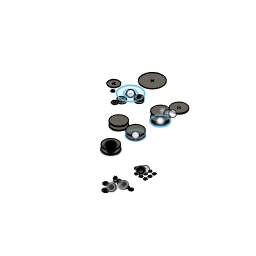
TwoBoardsThroghPlaneWith30mmHole v1 (Autodesk Fusion 360 design; units mm, degrees)
description: Spur Gear; Module: 2.0; Num Teeth: 16; Pressure Angle: 20.0; Backlash: 0.10 mm
Autodesk Fusion 360 part; units mm, degrees
(part 1 of 2)
sketch "Esquisse1" plane through (0, 0, 0) normal (0, 0, 1) x (1, 0, 0)
  circle A0 centre (0, 0) radius 70
  circle A1 centre (0, 0) radius 15
  dimension "d1" = 140
  dimension "d2" = 30
  constraint coincident A0.centre A1.centre
  constraint concentric A0 A1
  measures "d1" diameter of A0
  measures "d2" diameter of A1
sketch "Esquisse1 (2)" plane through (0, 0, 0) normal (0, 0, 1) x (1, 0, 0) in component "Spur Gear (16 teeth)"
  circle A0 centre (0, 0) radius 13.5492
  circle A1 centre (0, 0) radius 3
extrude "Extrusion1" add sketch "Esquisse1 (2)" along normal blind 2 contours A0 picked at (9.971186, -0.822177) makes body 1 in component "Spur Gear (16 teeth)"
sketch "Esquisse2" plane through (0, 0, 0) normal (0, 0, 1) x (1, 0, 0) in component "Spur Gear (16 teeth)"
  spline S0 degree 5 poles (14.941691, -1.673189) (14.950383, -1.674156) (14.967781, -1.675842) (14.993916, -1.677627) (15.028836, -1.678593) (15.072593, -1.677865) (15.116432, -1.675738) (15.160331, -1.672743) (15.204269, -1.669272) (15.248236, -1.665474) (15.292225, -1.661337) (15.336235, -1.656753) (15.380265, -1.651581) (15.424315, -1.645727) (15.468381, -1.639187) (15.512461, -1.632014) (15.556549, -1.624291) (15.600641, -1.616107) (15.644735, -1.607524) (15.688827, -1.598564) (15.732916, -1.589223) (15.777, -1.579481) (15.821079, -1.569317) (15.865151, -1.558721) (15.909214, -1.547697) (15.953267, -1.536261) (15.997307, -1.524432) (16.041334, -1.512231) (16.085345, -1.49967) (16.129338, -1.486758) (16.173313, -1.473495) (16.217269, -1.459883) (16.261203, -1.44592) (16.305115, -1.431607) (16.349004, -1.416949) (16.392868, -1.401951) (16.436706, -1.386619) (16.480518, -1.37096) (16.5243, -1.354979) (16.568053, -1.338679) (16.611776, -1.322063) (16.655467, -1.305134) (16.699125, -1.287892) (16.742749, -1.270341) (16.786339, -1.252484) (16.829892, -1.234323) (16.873409, -1.215861) (16.916887, -1.197102) (16.960326, -1.178048) (17.003726, -1.158702) (17.047084, -1.139066) (17.090401, -1.119141) (17.133674, -1.09893) (17.176904, -1.078435) (17.220089, -1.057658) (17.263228, -1.036601) (17.30632, -1.015266) (17.349365, -0.993655) (17.392361, -0.97177) (17.435308, -0.949612) (17.478204, -0.927183) (17.52105, -0.904486) (17.563844, -0.881521) (17.606585, -0.858289) (17.649272, -0.834794) (17.691904, -0.811036) (17.73448, -0.787018) (17.776999, -0.762741) (17.81946, -0.738205) (17.861864, -0.713414) (17.904209, -0.688366) (17.938038, -0.668124) (17.963384, -0.652828) (17.98027, -0.642579) (17.988709, -0.637443) knots 0 0 0 0 0 0 0.01428571 0.02857143 0.04285714 0.05714286 0.07142857 0.08571429 0.1 0.11428571 0.12857143 0.14285714 0.15714286 0.17142857 0.18571429 0.2 0.21428571 0.22857143 0.24285714 0.25714286 0.27142857 0.28571429 0.3 0.31428571 0.32857143 0.34285714 0.35714286 0.37142857 0.38571429 0.4 0.41428571 0.42857143 0.44285714 0.45714286 0.47142857 0.48571429 0.5 0.51428571 0.52857143 0.54285714 0.55714286 0.57142857 0.58571429 0.6 0.61428571 0.62857143 0.64285714 0.65714286 0.67142857 0.68571429 0.7 0.71428571 0.72857143 0.74285714 0.75714286 0.77142857 0.78571429 0.8 0.81428571 0.82857143 0.84285714 0.85714286 0.87142857 0.88571429 0.9 0.91428571 0.92857143 0.94285714 0.95714286 0.97142857 0.98571429 1 1 1 1 1 1
  spline S1 degree 5 poles (14.941691, 1.673189) (14.950383, 1.674156) (14.967781, 1.675842) (14.993916, 1.677627) (15.028836, 1.678593) (15.072593, 1.677865) (15.116432, 1.675738) (15.160331, 1.672743) (15.204269, 1.669272) (15.248236, 1.665474) (15.292225, 1.661337) (15.336235, 1.656753) (15.380265, 1.651581) (15.424315, 1.645727) (15.468381, 1.639187) (15.512461, 1.632014) (15.556549, 1.624291) (15.600641, 1.616107) (15.644735, 1.607524) (15.688827, 1.598564) (15.732916, 1.589223) (15.777, 1.579481) (15.821079, 1.569317) (15.865151, 1.558721) (15.909214, 1.547697) (15.953267, 1.536261) (15.997307, 1.524432) (16.041334, 1.512231) (16.085345, 1.49967) (16.129338, 1.486758) (16.173313, 1.473495) (16.217269, 1.459883) (16.261203, 1.44592) (16.305115, 1.431607) (16.349004, 1.416949) (16.392868, 1.401951) (16.436706, 1.386619) (16.480518, 1.37096) (16.5243, 1.354979) (16.568053, 1.338679) (16.611776, 1.322063) (16.655467, 1.305134) (16.699125, 1.287892) (16.742749, 1.270341) (16.786339, 1.252484) (16.829892, 1.234323) (16.873409, 1.215861) (16.916887, 1.197102) (16.960326, 1.178048) (17.003726, 1.158702) (17.047084, 1.139066) (17.090401, 1.119141) (17.133674, 1.09893) (17.176904, 1.078435) (17.220089, 1.057658) (17.263228, 1.036601) (17.30632, 1.015266) (17.349365, 0.993655) (17.392361, 0.97177) (17.435308, 0.949612) (17.478204, 0.927183) (17.52105, 0.904486) (17.563844, 0.881521) (17.606585, 0.858289) (17.649272, 0.834794) (17.691904, 0.811036) (17.73448, 0.787018) (17.776999, 0.762741) (17.81946, 0.738205) (17.861864, 0.713414) (17.904209, 0.688366) (17.938038, 0.668124) (17.963384, 0.652828) (17.98027, 0.642579) (17.988709, 0.637443) knots 0 0 0 0 0 0 0.01428571 0.02857143 0.04285714 0.05714286 0.07142857 0.08571429 0.1 0.11428571 0.12857143 0.14285714 0.15714286 0.17142857 0.18571429 0.2 0.21428571 0.22857143 0.24285714 0.25714286 0.27142857 0.28571429 0.3 0.31428571 0.32857143 0.34285714 0.35714286 0.37142857 0.38571429 0.4 0.41428571 0.42857143 0.44285714 0.45714286 0.47142857 0.48571429 0.5 0.51428571 0.52857143 0.54285714 0.55714286 0.57142857 0.58571429 0.6 0.61428571 0.62857143 0.64285714 0.65714286 0.67142857 0.68571429 0.7 0.71428571 0.72857143 0.74285714 0.75714286 0.77142857 0.78571429 0.8 0.81428571 0.82857143 0.84285714 0.85714286 0.87142857 0.88571429 0.9 0.91428571 0.92857143 0.94285714 0.95714286 0.97142857 0.98571429 1 1 1 1 1 1
  arc A0 (17.988709, -0.637443) -> (17.988709, 0.637443) centre (0, 0) ccw
  line L0 (13.455101, -1.507832) -> (14.941691, -1.673189)
  line L1 (13.455101, 1.507832) -> (14.941691, 1.673189)
  line L2 (13.455101, -1.507832) -> (13.455101, 1.507832)
  point P0 (15.154794, -1.673023)
  point P1 (15.370045, -1.652674)
  point P2 (15.586599, -1.618655)
  point P3 (15.804096, -1.573176)
  point P4 (16.022282, -1.517464)
  point P5 (16.240956, -1.45231)
  point P6 (16.459937, -1.378274)
  point P7 (16.679063, -1.295774)
  point P8 (16.898182, -1.205133)
  point P9 (17.117147, -1.106609)
  point P10 (17.335819, -1.000414)
  point P11 (17.554059, -0.886724)
  point P12 (17.771733, -0.76569)
  point P13 (15.154794, 1.673023)
  point P14 (15.370045, 1.652674)
  point P15 (15.586599, 1.618655)
  point P16 (15.804096, 1.573176)
  point P17 (16.022282, 1.517464)
  point P18 (16.240956, 1.45231)
  point P19 (16.459937, 1.378274)
  point P20 (16.679063, 1.295774)
  point P21 (16.898182, 1.205133)
  point P22 (17.117147, 1.106609)
  point P23 (17.335819, 1.000414)
  point P24 (17.554059, 0.886724)
  point P25 (17.771733, 0.76569)
extrude "Extrusion2" add sketch "Esquisse2" along normal blind 2 contours S0 S1 A0 L0 L1 L2 picked at (14.446161, -0.502611) bodies 1 in component "Spur Gear (16 teeth)"
fillet "Congé1" radius 1.1 2 edges at (13.464916, -1.508924, 1) (13.464916, 1.508924, 1) on bodies 1 in component "Spur Gear (16 teeth)"
pattern_circular "Réseau C1" count 16 over 360 about axis through (0, 0, 0) along (0, 0, 1) of "Extrusion2", "Congé1" in component "Spur Gear (16 teeth)"
sketch "Esquisse3" plane through (0, 0, 0) normal (0, 0, 1) x (1, 0, 0) in component "Spur Gear (16 teeth)"
  circle A0 centre (0, 0) radius 16 construction
sketch "Esquisse2 (2)" plane through (0, 0, 0) normal (0, 0, 1) x (1, 0, 0)
  line L0 (5, 2.886751) -> (0, 5.773503)
  line L1 (0, 5.773503) -> (-5, 2.886751)
  line L2 (-5, 2.886751) -> (-5, -2.886751)
  line L3 (-5, -2.886751) -> (0, -5.773503)
  line L4 (0, -5.773503) -> (5, -2.886751)
  line L5 (5, -2.886751) -> (5, 2.886751)
  line L6 (0, 6.062178) -> (-5.25, 3.031089)
  line L7 (-5.25, 3.031089) -> (-5.25, -3.031089)
  line L8 (-5.25, -3.031089) -> (0, -6.062178)
  line L9 (0, -6.062178) -> (5.25, -3.031089)
  line L10 (5.25, -3.031089) -> (5.25, 3.031089)
  line L11 (5.25, 3.031089) -> (0, 6.062178)
  dimension "d11" = 5
  dimension "d30" = 0.25
  measures "d11" distance of origin L5
extrude "Extrusion1'" add sketch "Esquisse2 (2)" along normal blind 5.25 separate body contours L0 L1 L2 L3 L4 L5 | L6 L7 L8 L9 L10 L11 picked at (1.666667, 0.96225) picked at (5.166667, -0.96225) makes body 2
extrude "Extrusion2'" add sketch "Esquisse1" along normal blind 8 separate body contours A0 | A1 picked at (51.406053, -3.477653) picked at (3.665259, 3.400864) makes body 3
sketch "Esquisse3 (2)" plane through (0, 0, 0) normal (0, 0, 1) x (1, 0, 0)
  line L0 (15, 0.000004) -> (12.135252, 8.816782)
  line L1 (12.135252, 8.816782) -> (4.635251, 14.265849)
  line L2 (4.635251, 14.265849) -> (-4.635259, 14.265846)
  line L3 (-4.635259, 14.265846) -> (-12.135257, 8.816775)
  line L4 (-12.135257, 8.816775) -> (-15, -0.000004)
  line L5 (-15, -0.000004) -> (-12.135252, -8.816782)
  line L6 (-12.135252, -8.816782) -> (-4.635251, -14.265849)
  line L7 (-4.635251, -14.265849) -> (4.635259, -14.265846)
  line L8 (4.635259, -14.265846) -> (12.135257, -8.816775)
  line L9 (12.135257, -8.816775) -> (15, 0.000004)
  line L10 (11, 0.000004) -> (8.899184, 6.465641)
  line L11 (8.899184, 6.465641) -> (3.399183, 10.461623)
  line L12 (3.399183, 10.461623) -> (-3.399191, 10.46162)
  line L13 (-3.399191, 10.46162) -> (-8.899189, 6.465634)
  line L14 (-8.899189, 6.465634) -> (-11, -0.000004)
  line L15 (-11, -0.000004) -> (-8.899184, -6.465641)
  line L16 (-8.899184, -6.465641) -> (-3.399183, -10.461623)
  line L17 (-3.399183, -10.461623) -> (3.399191, -10.46162)
  line L18 (3.399191, -10.46162) -> (8.899189, -6.465634)
  line L19 (8.899189, -6.465634) -> (11, 0.000004)
  line L20 (8.899184, 6.465641) -> (12.135252, 8.816782)
  line L21 (11, 0.000004) -> (15, 0.000004)
  line L22 (8.899189, -6.465634) -> (12.135257, -8.816775)
  line L23 (3.399191, -10.46162) -> (4.635259, -14.265846)
  line L24 (-3.399183, -10.461623) -> (-4.635251, -14.265849)
  line L25 (-8.899184, -6.465641) -> (-12.135252, -8.816782)
  line L26 (-11, -0.000004) -> (-15, -0.000004) construction
  line L27 (-8.899189, 6.465634) -> (-12.135257, 8.816775)
  line L28 (-3.399191, 10.46162) -> (-4.635259, 14.265846)
  line L29 (3.399183, 10.461623) -> (4.635251, 14.265849)
  circle A0 centre (-13.5, -0.000002) radius 1.5
  circle A1 centre (-11, -0.000004) radius 1.5 construction
  line L30 (-13.5, -0.000002) -> (-13.499999, 1.499998)
  line L31 (-13.5, -0.000002) -> (-13.500001, -1.500002)
  line L32 (-13.500001, -1.500002) -> (-11.000001, -1.500004)
  line L33 (-13.499999, 1.499998) -> (-10.999999, 1.499996)
  line L34 (-11.000001, -1.500004) -> (-10.51262, -1.500005)
  line L35 (-10.999999, 1.499996) -> (-11, -0.000004) construction
  line L36 (-10.999999, 1.499996) -> (-10.512621, 1.499995)
  line L37 (-11, -0.000004) -> (-11.000001, -1.500004) construction
  circle A2 centre (0, 0) radius 3
  dimension "d17" = 15
  dimension "d18" = 11
  dimension "d19" = 3
  dimension "d20" = 3
  dimension "d34" = 6
  constraint coincident A2.centre origin
  constraint horizontal L21
  constraint perpendicular L26 L30
  constraint perpendicular L26 L31
  constraint tangent A1 L32
  constraint tangent A1 L33
  constraint perpendicular L30 L33
  constraint tangent A1 L34
  constraint tangent A1 L36
  measures "d19" diameter of A0
  measures "d20" diameter of A1
  measures "d34" diameter of A2
extrude "Extrusion3" add sketch "Esquisse3 (2)" along normal blind 4 separate body contours L10 L11 L12 L13 L14 L15 L16 L17 L18 L19 | A2 picked at (-0.074733, 7.971618) picked at (-1.159118, 0.582926) makes body 4
extrude "Extrusion4" add sketch "Esquisse3 (2)" along normal blind 4 separate body contours L4 L5 A0 L30 L31 | L14 L15 A0 L32 L33 L34 L36 | A0 L30 L31 picked at (-14.404508, 0.29389) picked at (-11.353586, 0.640863) picked at (-13.428843, -0.994913) makes body 5
pattern_circular "Réseau C1'" count 10 over 360 about axis through (0, 0, 1.75) along (0, 0, 1) of bodies 5 makes body 6 at (-10.247547, -7.445282, 0) makes body 7 at (-3.914213, -12.046717, 0) makes body 8 at (3.914218, -12.046715, 0) makes body 9 at (10.24755, -7.445278, 0) makes body 10 at (12.666667, 0.000003, 0) makes body 11 at (10.247547, 7.445282, 0) makes body 12 at (3.914213, 12.046717, 0) makes body 13 at (-3.914218, 12.046715, 0) makes body 14 at (-10.24755, 7.445278, 0)
combine "Combiner1" operation add target body 12 tool bodies 11 10 9 8 4 7 6 5 14 13
move_body "Déplacer1" bodies 12 to x (1, 0, 0) y (0, 1, 0) z (0, 0, 1) at (0, 0, 4)
copy_body "Copier/Coller des corps1" bodies 12 makes body 15
move_body "Déplacer2" bodies 15 to x (1, 0, 0) y (0, 1, 0) z (0, 0, 1) at (0, 0, 16)
copy_body "Copier/Coller des corps2" bodies 12 makes body 16
move_body "Déplacer3" bodies 16 to x (1, 0, 0) y (0, 1, 0) z (0, 0, 1) at (350, 0, 0)
combine "Combiner2" operation cut target body 3 tool bodies 12 2
extrude "Extrusion5" cut sketch "Esquisse3 (2)" along normal blind 200 contours A2 picked at (-1.159118, 0.582926) bodies 15
sketch "Esquisse4" plane through (0, 0, 0) normal (0, 0, 1) x (1, 0, 0)
  circle A0 centre (350, 0) radius 15
  circle A1 centre (350, 0) radius 3
  dimension "d40" = 30
  dimension "d41" = 6
  constraint concentric A0 A1
  measures "d40" diameter of A0
  measures "d41" diameter of A1
extrude "Extrusion6" cut sketch "Esquisse4" along normal blind 20 contours A1 picked at (348.536266, 0.680173) bodies 16
pattern_linear "Réseau R1" count 3 spacing 45 along (1, 0, 0) count 3 spacing 45 along (0, -1, 0) of bodies 16 makes body 17 at (387.411364, 2.449965, 8) makes body 18 at (432.411364, 2.449965, 8) makes body 19 at (342.411364, -42.550035, 4) makes body 20 at (387.411364, -42.550035, 4) makes body 21 at (432.411364, -42.550035, 4) makes body 22 at (342.411364, -87.550035, 8) makes body 23 at (387.411364, -87.550035, 8) makes body 24 at (432.411364, -87.550035, 8)
sketch "Esquisse5" plane through (0, 0, 0) normal (0, 0, 1) x (1, 0, 0)
extrude "Extrusion7" add sketch "Esquisse4" along normal blind 2 separate body contours A0 picked at (360.932985, -0.894254) makes body 25
extrude "Extrusion8" add sketch "Esquisse4" along normal blind 6 separate body contours A0 picked at (360.932985, -0.894254) makes body 26
move_body "Déplacer4" bodies 26 to x (1, 0, 0) y (0, 1, 0) z (0, 0, 1) at (0, 0, 8)
extrude "Extrusion9" add 1 faces at (342.411364, -42.550035, 8) along direction (0, 0, 1) blind 6 on bodies 19 bodies 19
sketch "Esquisse6" plane through (0, 0, 14) normal (0, 0, 1) x (-1, 0, 0)
  circle A0 centre (-350, 45) radius 3
  arc A1 (-360.040052, 54.148624) -> (-361.385255, 54.361685) centre (-360.921731, 52.935099) ccw
  line L0 (-361.385255, 54.361685) -> (-362.135257, 53.816775)
  line L1 (-362.135257, 53.816775) -> (-362.421731, 52.935101)
  arc A2 (-362.421731, 52.935101) -> (-361.80341, 51.721575) centre (-360.921731, 52.935099) ccw
  line L2 (-361.80341, 51.721575) -> (-359.386569, 49.965633)
  line L3 (-359.386569, 49.965633) -> (-360.512621, 46.499995)
  line L4 (-360.512621, 46.499995) -> (-363.499999, 46.499998)
  arc A3 (-363.499999, 46.499998) -> (-364.713525, 45.881677) centre (-363.5, 44.999998) ccw
  line L5 (-364.713525, 45.881677) -> (-365, 44.999996)
  line L6 (-365, 44.999996) -> (-364.713526, 44.118321)
  arc A4 (-364.713526, 44.118321) -> (-363.500001, 43.499998) centre (-363.5, 44.999998) ccw
  line L7 (-363.500001, 43.499998) -> (-360.51262, 43.499995)
  line L8 (-360.51262, 43.499995) -> (-359.386564, 40.034358)
  line L9 (-359.386564, 40.034358) -> (-361.803405, 38.278424)
  arc A5 (-361.803405, 38.278424) -> (-362.421728, 37.064899) centre (-360.921728, 37.064898) ccw
  line L10 (-362.421728, 37.064899) -> (-362.135252, 36.183218)
  line L11 (-362.135252, 36.183218) -> (-361.385255, 35.638313)
  arc A6 (-361.385255, 35.638313) -> (-360.040052, 35.851371) centre (-360.921728, 37.064898) ccw
  line L12 (-360.040052, 35.851371) -> (-357.623207, 37.607308)
  line L13 (-357.623207, 37.607308) -> (-354.675159, 35.465427)
  line L14 (-354.675159, 35.465427) -> (-355.598312, 32.624263)
  arc A7 (-355.598312, 32.624263) -> (-355.385254, 31.27906) centre (-354.171728, 32.160736) ccw
  line L15 (-355.385254, 31.27906) -> (-354.635251, 30.734151)
  line L16 (-354.635251, 30.734151) -> (-353.708203, 30.734151)
  arc A8 (-353.708203, 30.734151) -> (-352.745143, 31.69721) centre (-354.171728, 32.160736) ccw
  line L17 (-352.745143, 31.69721) -> (-351.821989, 34.538378)
  line L18 (-351.821989, 34.538378) -> (-348.178002, 34.538379)
  line L19 (-348.178002, 34.538379) -> (-347.254854, 31.697213)
  arc A9 (-347.254854, 31.697213) -> (-346.291796, 30.734153) centre (-345.828269, 32.160738) ccw
  line L20 (-346.291796, 30.734153) -> (-345.364741, 30.734154)
  line L21 (-345.364741, 30.734154) -> (-344.614744, 31.279059)
  arc A10 (-344.614744, 31.279059) -> (-344.401683, 32.624262) centre (-345.828269, 32.160738) ccw
  line L22 (-344.401683, 32.624262) -> (-345.324833, 35.465432)
  line L23 (-345.324833, 35.465432) -> (-342.376786, 37.607315)
  line L24 (-342.376786, 37.607315) -> (-339.959948, 35.851376)
  arc A11 (-339.959948, 35.851376) -> (-338.614745, 35.638315) centre (-339.078269, 37.064901) ccw
  line L25 (-338.614745, 35.638315) -> (-337.864743, 36.183225)
  line L26 (-337.864743, 36.183225) -> (-337.578269, 37.064899)
  arc A12 (-337.578269, 37.064899) -> (-338.19659, 38.278425) centre (-339.078269, 37.064901) ccw
  line L27 (-338.19659, 38.278425) -> (-340.613431, 40.034367)
  line L28 (-340.613431, 40.034367) -> (-339.487379, 43.500005)
  line L29 (-339.487379, 43.500005) -> (-336.500001, 43.500002)
  arc A13 (-336.500001, 43.500002) -> (-335.286475, 44.118323) centre (-336.5, 45.000002) ccw
  line L30 (-335.286475, 44.118323) -> (-335, 45.000004)
  line L31 (-335, 45.000004) -> (-335.286474, 45.881679)
  arc A14 (-335.286474, 45.881679) -> (-336.499999, 46.500002) centre (-336.5, 45.000002) ccw
  line L32 (-336.499999, 46.500002) -> (-339.48738, 46.500005)
  line L33 (-339.48738, 46.500005) -> (-340.613436, 49.965642)
  line L34 (-340.613436, 49.965642) -> (-338.196595, 51.721576)
  arc A15 (-338.196595, 51.721576) -> (-337.578272, 52.935101) centre (-339.078272, 52.935102) ccw
  line L35 (-337.578272, 52.935101) -> (-337.864748, 53.816782)
  line L36 (-337.864748, 53.816782) -> (-338.614745, 54.361687)
  arc A16 (-338.614745, 54.361687) -> (-339.959948, 54.148629) centre (-339.078272, 52.935102) ccw
  line L37 (-339.959948, 54.148629) -> (-342.376793, 52.392692)
  line L38 (-342.376793, 52.392692) -> (-345.324841, 54.534573)
  line L39 (-345.324841, 54.534573) -> (-344.401688, 57.375737)
  arc A17 (-344.401688, 57.375737) -> (-344.614746, 58.72094) centre (-345.828272, 57.839264) ccw
  line L40 (-344.614746, 58.72094) -> (-345.364749, 59.265849)
  line L41 (-345.364749, 59.265849) -> (-346.291797, 59.265849)
  arc A18 (-346.291797, 59.265849) -> (-347.254857, 58.30279) centre (-345.828272, 57.839264) ccw
  line L42 (-347.254857, 58.30279) -> (-348.178011, 55.461622)
  line L43 (-348.178011, 55.461622) -> (-351.821998, 55.461621)
  line L44 (-351.821998, 55.461621) -> (-352.745146, 58.302787)
  arc A19 (-352.745146, 58.302787) -> (-353.708204, 59.265847) centre (-354.171731, 57.839262) ccw
  line L45 (-353.708204, 59.265847) -> (-354.635259, 59.265846)
  line L46 (-354.635259, 59.265846) -> (-355.385256, 58.720941)
  arc A20 (-355.385256, 58.720941) -> (-355.598317, 57.375738) centre (-354.171731, 57.839262) ccw
  line L47 (-355.598317, 57.375738) -> (-354.675167, 54.534568)
  line L48 (-354.675167, 54.534568) -> (-357.623214, 52.392685)
  line L49 (-357.623214, 52.392685) -> (-360.040052, 54.148624)
  circle A21 centre (-350, 45) radius 1.414218
  line L50 (-350, 45) -> (-349.999995, 34.538378) construction
  line L51 (-352.9977, 44.882561) -> (-360.51262, 44.882569) construction
  circle A22 centre (-356.75516, 44.882565) radius 2.5
  circle A23 centre (-349.882565, 38.24484) radius 2.5
  circle A24 centre (-343.24484, 45.117435) radius 2.5
  circle A25 centre (-350.117435, 51.75516) radius 2.5
  circle A26 centre (-356.75516, 44.882565) radius 1.5
  circle A27 centre (-349.882565, 38.24484) radius 1.5
  circle A28 centre (-343.24484, 45.117435) radius 1.5
  circle A29 centre (-350.117435, 51.75516) radius 1.5
  dimension "d57" = 5
  dimension "d59" = 360
  dimension "d62" = 3
  dimension "d64" = 360
  constraint concentric A0 A21
  constraint coincident A0.centre A21.centre
  constraint parallel L7 L51
  constraint concentric A22 A26
  measures "d57" diameter of A22
  measures "d62" diameter of A26
extrude "Extrusion10" cut sketch "Esquisse6" against normal blind 8 contours A22 | A23 | A24 | A25 | A26 | A27 | A28 | A29 picked at (-357.11413, 42.751658) picked at (-350.241535, 36.113933) picked at (-343.60381, 42.986528) picked at (-350.476405, 49.624253) picked at (-356.443415, 45.707365) picked at (-349.57082, 39.069639) picked at (-342.933095, 45.942234) picked at (-349.80569, 52.57996) bodies 19
copy_body "Copier/Coller des corps3" bodies 19 makes body 27
move_body "Déplacer5" bodies 27 to x (1, 0, 0) y (0, 1, 0) z (0, 0, 1) at (-45, 0, 0)
extrude "Extrusion11" add sketch "Esquisse6" against normal blind 10 contours A22 | A23 | A24 | A25 picked at (-357.11413, 42.751658) picked at (-350.241535, 36.113933) picked at (-343.60381, 42.986528) picked at (-350.476405, 49.624253) bodies 19
sketch "Esquisse7" plane through (0, 0, 0) normal (0, 1, 0) x (1, 0, 0)
sketch "Esquisse8" plane through (0, 0, 0) normal (0, 0, 1) x (1, 0, 0)
  circle A0 centre (375.003002, -250.002557) radius 15
  line L0 (375.003002, -250.002557) -> (375.003002, -235.002557)
  circle A1 centre (375.003004, -239.052557) radius 4.05
  circle A2 centre (364.588934, -246.618819) radius 4.05
  circle A3 centre (368.566753, -258.861292) radius 4.05
  circle A4 centre (381.43925, -258.861294) radius 4.05
  circle A5 centre (385.417072, -246.618822) radius 4.05
  circle A6 centre (375.003002, -250.002557) radius 17.5
  circle A7 centre (375.003002, -250.002557) radius 1
  line L1 (375.003004, -239.052557) -> (377.003004, -239.052557)
  line L2 (377.003004, -239.052557) -> (377.003004, -235.002557)
  line L3 (377.003004, -235.002557) -> (375.003004, -235.002557)
  line L4 (375.003004, -235.002557) -> (375.003004, -239.052557)
  line L5 (375.003004, -239.052557) -> (373.003004, -239.052557)
  line L6 (373.003004, -239.052557) -> (373.003004, -235.002557)
  line L7 (373.003004, -235.002557) -> (375.003004, -235.002557)
  line L8 (375.003004, -235.002557) -> (375.003004, -239.052557)
  circle A8 centre (375.003004, -239.052557) radius 1
  dimension "d70" = 30
  dimension "d71" = 8.1
  dimension "d73" = 360
  dimension "d74" = 35
  dimension "d75" = 2
  dimension "d83" = 2
  dimension "d84" = 2
  dimension "d85" = 2
  constraint vertical L0
  constraint concentric A0 A6
  constraint concentric A0 A7
  constraint horizontal L1
  constraint vertical L2
  constraint horizontal L3
  constraint vertical L4
  constraint horizontal L5
  constraint vertical L6
  constraint horizontal L7
  constraint vertical L8
  constraint concentric A1 A8
  measures "d70" diameter of A0
  measures "d71" diameter of A1
  measures "d74" diameter of A6
  measures "d75" diameter of A7
  measures "d85" diameter of A8
extrude "Extrusion12" add sketch "Esquisse8" along normal blind 3 separate body contours A0 A1 L2 L6 | A0 A1 L2 | A0 L2 L3 | A0 A1 L6 | A0 L6 L7 | A6 picked at (372.30825, -246.240467) picked at (376.846299, -235.323319) picked at (376.781519, -235.067059) picked at (373.159709, -235.323319) picked at (373.224489, -235.067059) picked at (375.003002, -233.368513) makes body 28
extrude "Extrusion13" add sketch "Esquisse8" along normal blind 3 separate body contours A0 A1 L2 L6 | A0 A1 L2 | A0 A1 L6 picked at (372.30825, -246.240467) picked at (376.846299, -235.323319) picked at (373.159709, -235.323319) makes body 29
move_body "Déplacer6" bodies 29 to x (1, 0, 0) y (0, 1, 0) z (0, 0, 1) at (0, 0, 1)
combine "Combiner3" operation cut target body 28 tool bodies 29
copy_body "Copier/Coller des corps4" bodies 28 makes body 30
move_body "Déplacer7" bodies 30 to x (1, 0, 0) y (0, 1, 0) z (0, 0, 1) at (40, 0, 0)
extrude "Extrusion14" add sketch "Esquisse8" along normal blind 1 separate body contours L0 A1 L1 L2 L4 L8 A8 | L0 A1 L4 L5 L6 L8 A8 picked at (376.588254, -237.660364) picked at (373.417754, -237.660364) makes body 31
pattern_circular "Réseau C2" count 5 over 360 about axis through (375.003002, -250.002557, 0) along (0, 0, 1) of bodies 31 makes body 32 at (363.754749, -244.680946, 0) makes body 33 at (366.465948, -259.055813, 0) makes body 34 at (380.975066, -260.919388, 0) makes body 35 at (387.230995, -247.696273, 0)
combine "Combiner4" operation add target body 28 tool bodies 31 32 33 34 35
move_body "Déplacer8" bodies 28 to x (1, 0, 0) y (0, 1, 0) z (0, 0, 1) at (80, 0, 0)
extrude "Extrusion15" add sketch "Esquisse8" along normal blind 20 separate body contours A0 A1 L2 L6 | A0 A1 L2 | A0 A1 L6 picked at (372.30825, -246.240467) picked at (376.846299, -235.323319) picked at (373.159709, -235.323319) makes body 36
extrude "Extrusion16" add sketch "Esquisse8" along normal blind 12 separate body contours A5 | A2 | A3 | A4 | L0 A1 L1 L2 L4 L8 A8 | L0 A1 L4 L5 L6 L8 A8 | L0 A1 L1 L2 A8 | L0 L1 L4 L8 A8 | L0 L4 L5 L8 A8 | L0 A1 L5 L6 A8 | L0 L1 A8 | L0 L5 A8 picked at (384.313397, -247.937122) picked at (365.008905, -247.746883) picked at (367.598711, -260.855074) picked at (380.311446, -258.763584) picked at (376.588254, -237.660364) picked at (373.417754, -237.660364) picked at (376.941849, -240.154906) picked at (375.401504, -238.520222) picked at (374.861654, -238.402785) picked at (373.048206, -240.136152) picked at (375.144352, -239.702328) picked at (374.955564, -239.715831) makes body 37 at (365.338366, -256.415884, 8) makes body 38 at (384.713797, -250.607294, 4) makes body 39 at (363.885659, -250.607291, 4) makes body 40 at (375.706279, -235.064085, 8) makes body 41 at (381.338281, -254.812553, 8)
extrude "Extrusion17" cut sketch "Esquisse8" along normal blind 8 contours A5 | A2 | A3 | A4 | L0 A1 L1 L2 L4 L8 A8 | L0 A1 L4 L5 L6 L8 A8 | L0 A1 L1 L2 A8 | L0 L1 L4 L8 A8 | L0 L4 L5 L8 A8 | L0 A1 L5 L6 A8 | L0 L1 A8 | L0 L5 A8 picked at (384.313397, -247.937122) picked at (365.008905, -247.746883) picked at (367.598711, -260.855074) picked at (380.311446, -258.763584) picked at (376.588254, -237.660364) picked at (373.417754, -237.660364) picked at (376.941849, -240.154906) picked at (375.401504, -238.520222) picked at (374.861654, -238.402785) picked at (373.048206, -240.136152) picked at (375.144352, -239.702328) picked at (374.955564, -239.715831) bodies 37 38 39 40 41
combine "Combiner5" operation add target body 40 tool bodies 38 39 37 41 36
move_body "Déplacer9" bodies 40 to x (1, 0, 0) y (0, 1, 0) z (0, 0, 1) at (-40, 0, 0)
extrude "Extrusion18" add sketch "Esquisse8" against normal blind 8 separate body contours A5 | A2 | A3 | A4 | L0 A1 L1 L2 L4 L8 A8 | L0 A1 L4 L5 L6 L8 A8 | L0 A1 L1 L2 A8 | L0 L1 L4 L8 A8 | L0 L4 L5 L8 A8 | L0 A1 L5 L6 A8 | L0 L1 A8 | L0 L5 A8 picked at (384.313397, -247.937122) picked at (365.008905, -247.746883) picked at (367.598711, -260.855074) picked at (380.311446, -258.763584) picked at (376.588254, -237.660364) picked at (373.417754, -237.660364) picked at (376.941849, -240.154906) picked at (375.401504, -238.520222) picked at (374.861654, -238.402785) picked at (373.048206, -240.136152) picked at (375.144352, -239.702328) picked at (374.955564, -239.715831) makes body 42 at (365.464273, -256.258002, -2.666667) makes body 43 at (381.338281, -262.910035, -2.666667) makes body 44 at (365.092526, -242.600251, -5.333333) makes body 45 at (385.920664, -242.600253, -5.333333) makes body 46 at (375.506596, -235.033988, -5.333333)
extrude "Extrusion19" add sketch "Esquisse8" along normal blind 28 contours A5 | A2 | A3 | A4 | L0 A1 L1 L2 L4 L8 A8 | L0 A1 L4 L5 L6 L8 A8 | L0 A1 L1 L2 A8 | L0 L1 L4 L8 A8 | L0 L4 L5 L8 A8 | L0 A1 L5 L6 A8 | L0 L1 A8 | L0 L5 A8 picked at (384.313397, -247.937122) picked at (365.008905, -247.746883) picked at (367.598711, -260.855074) picked at (380.311446, -258.763584) picked at (376.588254, -237.660364) picked at (373.417754, -237.660364) picked at (376.941849, -240.154906) picked at (375.401504, -238.520222) picked at (374.861654, -238.402785) picked at (373.048206, -240.136152) picked at (375.144352, -239.702328) picked at (374.955564, -239.715831) bodies 42 43 44 45 46
extrude "Extrusion20" add sketch "Esquisse8" along normal blind 20 separate body contours A0 A1 L2 L6 | A0 A1 L2 | A0 A1 L6 picked at (372.30825, -246.240467) picked at (376.846299, -235.323319) picked at (373.159709, -235.323319) makes body 47
combine "Combiner6" operation add target body 47 tool bodies 46 44 42 43 45
move_body "Déplacer10" bodies 47 to x (1, 0, 0) y (0, 1, 0) z (0, 0, 1) at (-80, 0, 0)
sketch "Esquisse9" plane through (0, 0, 0) normal (0, 0, 1) x (1, 0, 0)
  circle A0 centre (375, -300) radius 4
  circle A1 centre (375, -300) radius 4.5
  circle A2 centre (375, -300) radius 6
  dimension "d114" = 8
  dimension "d115" = 9
  dimension "d116" = 12
  constraint concentric A0 A1
  constraint concentric A1 A2
  measures "d114" diameter of A0
  measures "d115" diameter of A1
  measures "d116" diameter of A2
extrude "Extrusion21" add sketch "Esquisse9" along normal blind 4 separate body contours A0 | A1 | A2 picked at (376.274097, -302.206801) picked at (373.821512, -304.158606) picked at (369.935463, -297.891897) makes body 48
extrude "Extrusion22" add sketch "Esquisse9" against normal blind 8 contours A0 picked at (376.274097, -302.206801) bodies 48
extrude "Extrusion23" add sketch "Esquisse9" along normal blind 12 contours A0 picked at (376.274097, -302.206801) bodies 48
sketch "Esquisse10" plane through (0, 0, 0) normal (0, 0, 1) x (1, 0, 0)
  circle A0 centre (375, -300) radius 4
  line L0 (379, -300) -> (377.5, -300)
  line L1 (377.5, -300) -> (377.5, -294.000004)
  line L2 (377.5, -300) -> (377.5, -306.000005)
  circle A1 centre (375, -300) radius 6
  point P0 (375, -300)
  dimension "d123" = 8
  dimension "d124" = 1.5
  dimension "d127" = 12
  constraint coincident P0 A0.centre
  constraint coincident A0 L0.start
  constraint horizontal L0
  constraint perpendicular L0 L1
  constraint perpendicular L0 L2
  measures "d123" diameter of A0
  measures "d124" distance of L0.start L0.end
  measures "d127" diameter of A1
extrude "Extrusion24" cut sketch "Esquisse10" along normal blind 40 and the other way blind 40 contours A0 L0 L1 | A0 L1 L2 A1 | A0 L0 L2 picked at (378.485172, -299.801702) picked at (378.227922, -295.767817) picked at (378.485172, -300.198298) bodies 48
sketch "Esquisse11" plane through (0, 0, 12) normal (0, 0, 1) x (-1, 0, 0)
  line L0 (-377.5, 303.122499) -> (-377.5, 296.877501)
  arc A0 (-377.5, 296.877501) -> (-377.5, 303.122499) centre (-375, 300) ccw
extrude "Extrusion25" add sketch "Esquisse11" along normal blind 20 separate body contours L0 A0 picked at (-376.036383, 301.040833) makes body 49
move_body "Déplacer11" bodies 49 to x (1, 0, 0) y (0, 1, 0) z (0, 0, 1) at (-40, -40, -20)
sketch "Esquisse12" plane through (0, 0, 12) normal (0, 0, 1) x (-1, 0, 0)
  arc A0 (-337.5, 336.877501) -> (-337.5, 343.122499) centre (-335, 340) ccw
  line L0 (-337.5, 343.122499) -> (-337.5, 336.877501)
  circle A1 centre (-346, 340) radius 15
  line L1 (-344.454163, 348.922465) -> (-339.045837, 345.799966)
  arc A2 (-339.045837, 345.799966) -> (-344.454163, 348.922465) centre (-340.5, 349.526279) ccw
  line L2 (-352.954163, 345.799966) -> (-347.545837, 348.922465)
  arc A3 (-347.545837, 348.922465) -> (-352.954163, 345.799966) centre (-351.5, 349.526279) ccw
  line L3 (-354.5, 336.877501) -> (-354.5, 343.122499)
  arc A4 (-354.5, 343.122499) -> (-354.5, 336.877501) centre (-357, 340) ccw
  line L4 (-347.545837, 331.077535) -> (-352.954163, 334.200034)
  arc A5 (-352.954163, 334.200034) -> (-347.545837, 331.077535) centre (-351.5, 330.473721) ccw
  line L5 (-339.045837, 334.200034) -> (-344.454163, 331.077535)
  arc A6 (-344.454163, 331.077535) -> (-339.045837, 334.200034) centre (-340.5, 330.473721) ccw
  line L6 (-341, 342.886751) -> (-346, 345.773503)
  line L7 (-346, 345.773503) -> (-351, 342.886751)
  line L8 (-351, 342.886751) -> (-351, 337.113249)
  line L9 (-351, 337.113249) -> (-346, 334.226497)
  line L10 (-346, 334.226497) -> (-341, 337.113249)
  line L11 (-341, 337.113249) -> (-341, 342.886751)
  circle A7 centre (-346, 340) radius 20
  circle A8 centre (-346, 340) radius 3
  circle A9 centre (-346, 340) radius 25
  point P0 (-346, 340)
  dimension "d137" = 30
  dimension "d139" = 360
  dimension "d140" = 5
  dimension "d141" = 40
  dimension "d146" = 6
  dimension "d153" = 50
  constraint coincident P0 A1.centre
  constraint concentric A1 A7
  measures "d137" diameter of A1
  measures "d140" distance of P0 L11
  measures "d141" diameter of A7
  measures "d146" diameter of A8
  measures "d153" diameter of A9
extrude "Extrusion26" add sketch "Esquisse12" along normal blind 3 separate body contours A7 picked at (-337.73106, 323.690545) makes body 50
extrude "Extrusion27" add sketch "Esquisse12" along normal blind 8 contours A1 | L6 L7 L8 L9 L10 L11 | A8 picked at (-353.333333, 339.03775) picked at (-341.666667, 340) picked at (-346.365341, 340.930874) bodies 50
extrude "Extrusion28" cut sketch "Esquisse12" along normal blind 8 contours A8 picked at (-346.365341, 340.930874) bodies 50
extrude "Extrusion29" cut sketch "Esquisse12" along normal blind 5 contours L6 L7 L8 L9 L10 L11 picked at (-341.666667, 340) bodies 50
extrude "Extrusion30" add sketch "Esquisse12" along normal blind 30 separate body contours A0 L0 | L1 A2 | L2 A3 | L3 A4 | L4 A5 | L5 A6 | A8 picked at (-335.449017, 339.046963) picked at (-339.567496, 350.234954) picked at (-351.98368, 350.592974) picked at (-359.664583, 340) picked at (-349.688213, 331.011333) picked at (-341.508844, 328.216463) picked at (-346.365341, 340.930874) makes body 51 at (344.014942, -342.249344, 32) makes body 52 at (332.832703, -336.638033, 22) makes body 53 at (355.719866, -343.789625, 32) makes body 54 at (347.739177, -350.888707, 32) makes body 55 at (336.742878, -331.846321, 22) makes body 56 at (350.413992, -326.623969, 32) makes body 57 at (336.742878, -348.153679, 32)
extrude "Extrusion31" add sketch "Esquisse12" 7 faces at (346.365341, -340.930874, 12) (339.538738, -348.81317, 12) (359.664583, -340, 12) (339.457749, -330.119943, 12) (350.535225, -351.978059, 12) (350.29807, -330.298266, 12) (336.036383, -341.040833, 12) along normal blind 4 separate body contours A0 L0 | L1 A2 | L2 A3 | L3 A4 | L4 A5 | L5 A6 | A1 | L6 L7 L8 L9 L10 L11 | A7 | A8 | A9 picked at (-335.449017, 339.046963) picked at (-339.567496, 350.234954) picked at (-351.98368, 350.592974) picked at (-359.664583, 340) picked at (-349.688213, 331.011333) picked at (-341.508844, 328.216463) picked at (-353.333333, 339.03775) picked at (-341.666667, 340) picked at (-337.73106, 323.690545) picked at (-346.365341, 340.930874) picked at (-322.834204, 337.764366) on bodies 51 52 53 54 55 56 57 makes body 58
combine "Combiner7" operation cut target body 58 tool bodies 51 56 57 52 55 53 54
move_body "Déplacer12" bodies 58 to x (1, 0, 0) y (0, 1, 0) z (0, 0, 1) at (0, -60, 0)
move_body "Déplacer13" bodies 48 to x (0, 0, -1) y (0, 1, 0) z (1, 0, 0) at (385.5, 0, 369.5)
pattern_linear "Réseau R2" count 6 spacing 15 along (0, -1, 0) of bodies 48 makes body 59 at (394.833333, -313.444994, -1.814629) makes body 60 at (394.833333, -328.444994, -1.814629) makes body 61 at (394.833333, -343.444994, -1.814629) makes body 62 at (394.833333, -358.444994, -1.814629) makes body 63 at (394.833333, -373.444994, -1.814629)
move_body "Déplacer14" bodies 50 to x (1, 0, 0) y (0, 1, 0) z (0, 0, 1) at (-60, 0, 0)
copy_body "Copier/Coller des corps5" bodies 15 makes body 64
move_body "Déplacer15" bodies 64 to x (1, 0, 0) y (0, 1, 0) z (0, 0, 1) at (0, 0, -15)
copy_body "Copier/Coller des corps6" bodies 3 makes body 65
move_body "Déplacer16" bodies 65 to x (1, 0, 0) y (0, 1, 0) z (0, 0, 1) at (0, 0, 9)
extrude "Extrusion32" add 1 faces at (-3.308389, 6.209278, 13) along direction (0, 0, 1) blind 4 on bodies 65 bodies 65
move_body "Déplacer17" bodies 65 to x (1, 0, 0) y (0, 1, 0) z (0, 0, 1) at (0, 0, 29)
move_body "Déplacer18" bodies 64 to x (1, 0, 0) y (0, 1, 0) z (0, 0, 1) at (0, 0, 30)
copy_body "Copier/Coller des corps7" bodies 15 makes body 66
move_body "Déplacer19" bodies 66 to x (1, 0, 0) y (0, 1, 0) z (0, 0, 1) at (0, 0, 11)
combine "Combiner8" operation add target body 66 tool bodies 64 65
sketch "Esquisse13" plane through (0, 0, 31) normal (0, 0, -1) x (1, 0, 0)
  circle A0 centre (0, 0) radius 3
  arc A1 (11.385255, 9.361685) -> (10.040052, 9.148624) centre (10.921731, 7.935099) ccw
  line L0 (10.040052, 9.148624) -> (7.623214, 7.392685)
  line L1 (7.623214, 7.392685) -> (4.675167, 9.534568)
  line L2 (4.675167, 9.534568) -> (5.598317, 12.375738)
  arc A2 (5.598317, 12.375738) -> (5.385256, 13.720941) centre (4.171731, 12.839262) ccw
  line L3 (5.385256, 13.720941) -> (4.635259, 14.265846)
  line L4 (4.635259, 14.265846) -> (3.708204, 14.265847)
  arc A3 (3.708204, 14.265847) -> (2.745146, 13.302787) centre (4.171731, 12.839262) ccw
  line L5 (2.745146, 13.302787) -> (1.821998, 10.461621)
  line L6 (1.821998, 10.461621) -> (-1.821989, 10.461622)
  line L7 (-1.821989, 10.461622) -> (-2.745143, 13.30279)
  arc A4 (-2.745143, 13.30279) -> (-3.708203, 14.265849) centre (-4.171728, 12.839264) ccw
  line L8 (-3.708203, 14.265849) -> (-4.635251, 14.265849)
  line L9 (-4.635251, 14.265849) -> (-5.385254, 13.72094)
  arc A5 (-5.385254, 13.72094) -> (-5.598312, 12.375737) centre (-4.171728, 12.839264) ccw
  line L10 (-5.598312, 12.375737) -> (-4.675159, 9.534573)
  line L11 (-4.675159, 9.534573) -> (-7.623207, 7.392692)
  line L12 (-7.623207, 7.392692) -> (-10.040052, 9.148629)
  arc A6 (-10.040052, 9.148629) -> (-11.385255, 9.361687) centre (-10.921728, 7.935102) ccw
  line L13 (-11.385255, 9.361687) -> (-12.135252, 8.816782)
  line L14 (-12.135252, 8.816782) -> (-12.421728, 7.935101)
  arc A7 (-12.421728, 7.935101) -> (-11.803405, 6.721576) centre (-10.921728, 7.935102) ccw
  line L15 (-11.803405, 6.721576) -> (-9.386564, 4.965642)
  line L16 (-9.386564, 4.965642) -> (-10.51262, 1.500005)
  line L17 (-10.51262, 1.500005) -> (-13.500001, 1.500002)
  arc A8 (-13.500001, 1.500002) -> (-14.713526, 0.881679) centre (-13.5, 0.000002) ccw
  line L18 (-14.713526, 0.881679) -> (-15, 0.000004)
  line L19 (-15, 0.000004) -> (-14.713525, -0.881677)
  arc A9 (-14.713525, -0.881677) -> (-13.499999, -1.499998) centre (-13.5, 0.000002) ccw
  line L20 (-13.499999, -1.499998) -> (-10.512621, -1.499995)
  line L21 (-10.512621, -1.499995) -> (-9.386569, -4.965633)
  line L22 (-9.386569, -4.965633) -> (-11.80341, -6.721575)
  arc A10 (-11.80341, -6.721575) -> (-12.421731, -7.935101) centre (-10.921731, -7.935099) ccw
  line L23 (-12.421731, -7.935101) -> (-12.135257, -8.816775)
  line L24 (-12.135257, -8.816775) -> (-11.385255, -9.361685)
  arc A11 (-11.385255, -9.361685) -> (-10.040052, -9.148624) centre (-10.921731, -7.935099) ccw
  line L25 (-10.040052, -9.148624) -> (-7.623214, -7.392685)
  line L26 (-7.623214, -7.392685) -> (-4.675167, -9.534568)
  line L27 (-4.675167, -9.534568) -> (-5.598317, -12.375738)
  arc A12 (-5.598317, -12.375738) -> (-5.385256, -13.720941) centre (-4.171731, -12.839262) ccw
  line L28 (-5.385256, -13.720941) -> (-4.635259, -14.265846)
  line L29 (-4.635259, -14.265846) -> (-3.708204, -14.265847)
  arc A13 (-3.708204, -14.265847) -> (-2.745146, -13.302787) centre (-4.171731, -12.839262) ccw
  line L30 (-2.745146, -13.302787) -> (-1.821998, -10.461621)
  line L31 (-1.821998, -10.461621) -> (1.821989, -10.461622)
  line L32 (1.821989, -10.461622) -> (2.745143, -13.30279)
  arc A14 (2.745143, -13.30279) -> (3.708203, -14.265849) centre (4.171728, -12.839264) ccw
  line L33 (3.708203, -14.265849) -> (4.635251, -14.265849)
  line L34 (4.635251, -14.265849) -> (5.385254, -13.72094)
  arc A15 (5.385254, -13.72094) -> (5.598312, -12.375737) centre (4.171728, -12.839264) ccw
  line L35 (5.598312, -12.375737) -> (4.675159, -9.534573)
  line L36 (4.675159, -9.534573) -> (7.623207, -7.392692)
  line L37 (7.623207, -7.392692) -> (10.040052, -9.148629)
  arc A16 (10.040052, -9.148629) -> (11.385255, -9.361687) centre (10.921728, -7.935102) ccw
  line L38 (11.385255, -9.361687) -> (12.135252, -8.816782)
  line L39 (12.135252, -8.816782) -> (12.421728, -7.935101)
  arc A17 (12.421728, -7.935101) -> (11.803405, -6.721576) centre (10.921728, -7.935102) ccw
  line L40 (11.803405, -6.721576) -> (9.386564, -4.965642)
  line L41 (9.386564, -4.965642) -> (10.51262, -1.500005)
  line L42 (10.51262, -1.500005) -> (13.500001, -1.500002)
  arc A18 (13.500001, -1.500002) -> (14.713526, -0.881679) centre (13.5, -0.000002) ccw
  line L43 (14.713526, -0.881679) -> (15, -0.000004)
  line L44 (15, -0.000004) -> (14.713525, 0.881677)
  arc A19 (14.713525, 0.881677) -> (13.499999, 1.499998) centre (13.5, -0.000002) ccw
  line L45 (13.499999, 1.499998) -> (10.512621, 1.499995)
  line L46 (10.512621, 1.499995) -> (9.386569, 4.965633)
  line L47 (9.386569, 4.965633) -> (11.80341, 6.721575)
  arc A20 (11.80341, 6.721575) -> (12.421731, 7.935101) centre (10.921731, 7.935099) ccw
  line L48 (12.421731, 7.935101) -> (12.135257, 8.816775)
  line L49 (12.135257, 8.816775) -> (11.385255, 9.361685)
  arc A21 (5.408105, 12.437541) -> (5.241131, 13.578441) centre (4.171731, 12.839262) ccw
  line L50 (5.241131, 13.578441) -> (4.570275, 14.065846)
  line L51 (4.570275, 14.065846) -> (3.741045, 14.065847)
  arc A22 (3.741045, 14.065847) -> (2.935357, 13.240983) centre (4.171731, 12.839262) ccw
  line L52 (2.935357, 13.240983) -> (1.967307, 10.261621)
  line L53 (1.967307, 10.261621) -> (-1.967297, 10.261622)
  line L54 (-1.967297, 10.261622) -> (-2.935354, 13.240987)
  arc A23 (-2.935354, 13.240987) -> (-3.741044, 14.065849) centre (-4.171728, 12.839264) ccw
  line L55 (-3.741044, 14.065849) -> (-4.570267, 14.065849)
  line L56 (-4.570267, 14.065849) -> (-5.241129, 13.57844)
  arc A24 (-5.241129, 13.57844) -> (-5.408101, 12.43754) centre (-4.171728, 12.839264) ccw
  line L57 (-5.408101, 12.43754) -> (-4.440045, 9.45818)
  line L58 (-4.440045, 9.45818) -> (-7.623207, 7.145479)
  line L59 (-7.623207, 7.145479) -> (-10.157608, 8.986825)
  arc A25 (-10.157608, 8.986825) -> (-11.294266, 9.18058) centre (-10.921728, 7.935102) ccw
  line L60 (-11.294266, 9.18058) -> (-11.965122, 8.693175)
  line L61 (-11.965122, 8.693175) -> (-12.221369, 7.904531)
  arc A26 (-12.221369, 7.904531) -> (-11.685848, 6.88338) centre (-10.921728, 7.935102) ccw
  line L62 (-11.685848, 6.88338) -> (-9.15145, 5.042035)
  line L63 (-9.15145, 5.042035) -> (-10.367311, 1.300005)
  line L64 (-10.367311, 1.300005) -> (-13.500001, 1.300002)
  arc A27 (-13.500001, 1.300002) -> (-14.533463, 0.788642) centre (-13.5, 0.000002) ccw
  line L65 (-14.533463, 0.788642) -> (-14.789708, 0.000004)
  line L66 (-14.789708, 0.000004) -> (-14.533462, -0.788641)
  arc A28 (-14.533462, -0.788641) -> (-13.499999, -1.299998) centre (-13.5, 0.000002) ccw
  line L67 (-13.499999, -1.299998) -> (-10.367313, -1.299995)
  line L68 (-10.367313, -1.299995) -> (-9.151455, -5.042027)
  line L69 (-9.151455, -5.042027) -> (-11.685852, -6.883378)
  arc A29 (-11.685852, -6.883378) -> (-12.221371, -7.90453) centre (-10.921731, -7.935099) ccw
  line L70 (-12.221371, -7.90453) -> (-11.965127, -8.693169)
  line L71 (-11.965127, -8.693169) -> (-11.294266, -9.180578)
  arc A30 (-11.294266, -9.180578) -> (-10.157609, -8.986821) centre (-10.921731, -7.935099) ccw
  line L72 (-10.157609, -8.986821) -> (-7.623214, -7.145472)
  line L73 (-7.623214, -7.145472) -> (-4.440053, -9.458175)
  line L74 (-4.440053, -9.458175) -> (-5.408105, -12.437541)
  arc A31 (-5.408105, -12.437541) -> (-5.241131, -13.578441) centre (-4.171731, -12.839262) ccw
  line L75 (-5.241131, -13.578441) -> (-4.570275, -14.065846)
  line L76 (-4.570275, -14.065846) -> (-3.741045, -14.065847)
  arc A32 (-3.741045, -14.065847) -> (-2.935357, -13.240983) centre (-4.171731, -12.839262) ccw
  line L77 (-2.935357, -13.240983) -> (-1.967307, -10.261621)
  line L78 (-1.967307, -10.261621) -> (1.967297, -10.261622)
  line L79 (1.967297, -10.261622) -> (2.935354, -13.240987)
  arc A33 (2.935354, -13.240987) -> (3.741044, -14.065849) centre (4.171728, -12.839264) ccw
  line L80 (3.741044, -14.065849) -> (4.570267, -14.065849)
  line L81 (4.570267, -14.065849) -> (5.241129, -13.57844)
  arc A34 (5.241129, -13.57844) -> (5.408101, -12.43754) centre (4.171728, -12.839264) ccw
  line L82 (5.408101, -12.43754) -> (4.440045, -9.45818)
  line L83 (4.440045, -9.45818) -> (7.623207, -7.145479)
  line L84 (7.623207, -7.145479) -> (10.157608, -8.986825)
  arc A35 (10.157608, -8.986825) -> (11.294266, -9.18058) centre (10.921728, -7.935102) ccw
  line L85 (11.294266, -9.18058) -> (11.965122, -8.693175)
  line L86 (11.965122, -8.693175) -> (12.221369, -7.904531)
  arc A36 (12.221369, -7.904531) -> (11.685848, -6.88338) centre (10.921728, -7.935102) ccw
  line L87 (11.685848, -6.88338) -> (9.15145, -5.042035)
  line L88 (9.15145, -5.042035) -> (10.367311, -1.300005)
  line L89 (10.367311, -1.300005) -> (13.500001, -1.300002)
  arc A37 (13.500001, -1.300002) -> (14.533463, -0.788642) centre (13.5, -0.000002) ccw
  line L90 (14.533463, -0.788642) -> (14.789708, -0.000004)
  line L91 (14.789708, -0.000004) -> (14.533462, 0.788641)
  arc A38 (14.533462, 0.788641) -> (13.499999, 1.299998) centre (13.5, -0.000002) ccw
  line L92 (13.499999, 1.299998) -> (10.367313, 1.299995)
  line L93 (10.367313, 1.299995) -> (9.151455, 5.042027)
  line L94 (9.151455, 5.042027) -> (11.685852, 6.883378)
  arc A39 (11.685852, 6.883378) -> (12.221371, 7.90453) centre (10.921731, 7.935099) ccw
  line L95 (12.221371, 7.90453) -> (11.965127, 8.693169)
  line L96 (11.965127, 8.693169) -> (11.294266, 9.180578)
  arc A40 (11.294266, 9.180578) -> (10.157609, 8.986821) centre (10.921731, 7.935099) ccw
  line L97 (10.157609, 8.986821) -> (7.623214, 7.145472)
  line L98 (7.623214, 7.145472) -> (4.440053, 9.458175)
  line L99 (4.440053, 9.458175) -> (5.408105, 12.437541)
  dimension "d184" = -0.2
extrude "Extrusion33" cut sketch "Esquisse13" against normal blind 7 contours A1 L0 L1 L2 A2 L3 L4 A3 L5 L6 L7 A4 L8 L9 A5 L10 L11 L12 A6 L13 L14 A7 L15 L16 L17 A8 L18 L19 A9 L20 L21 L22 A10 L23 L24 A11 L25 L26 L27 A12 L28 L29 A13 L30 L31 L32 A14 L33 L34 A15 L35 L36 L37 A16 L38 L39 A17 L40 L41 L42 A18 L43 L44 A19 L45 L46 L47 A20 L48 L49 picked at (-5.57947, 8.712744) bodies 66
sketch "Esquisse14" plane through (0, 0, 0) normal (0, 0, 1) x (1, 0, 0)
  circle A0 centre (0, 250) radius 70
  circle A1 centre (0, 250) radius 15
  circle A2 centre (0, 250) radius 5
  circle A3 centre (0, 250) radius 12
  dimension "d187" = 140
  dimension "d188" = 30
  dimension "d189" = 10
  dimension "d209" = -3
  constraint concentric A0 A1
  constraint concentric A0 A2
  measures "d187" diameter of A0
  measures "d188" diameter of A1
  measures "d189" diameter of A2
extrude "Extrusion34" add sketch "Esquisse14" along normal blind 8 separate body contours A0 | A1 | A2 | A3 picked at (51.406053, 246.522347) picked at (13.899477, 248.65862) picked at (1.57507, 251.443376) picked at (-9.603375, 249.155427) makes body 67
move_body "Déplacer20" bodies 67 to x (1, 0, 0) y (0, 1, 0) z (0, 0, 1) at (0, 0, 8)
extrude "Extrusion35" add sketch "Esquisse14" along normal blind 8 separate body contours A0 | A1 | A2 | A3 picked at (51.406053, 246.522347) picked at (13.899477, 248.65862) picked at (1.57507, 251.443376) picked at (-9.603375, 249.155427) makes body 68
move_body "Déplacer21" bodies 67 to x (1, 0, 0) y (0, 1, 0) z (0, 0, 1) at (0, 0, 3)
extrude "Extrusion36" add sketch "Esquisse14" along normal blind 11 contours A1 | A3 picked at (13.899477, 248.65862) picked at (-9.603375, 249.155427) bodies 68
extrude "Extrusion37" add sketch "Esquisse14" along normal blind 11 separate body contours A2 picked at (1.57507, 251.443376) makes body 69
combine "Combiner9" operation add target body 69 tool bodies 67
move_body "Déplacer22" bodies 69 to x (1, 0, 0) y (0, 1, 0) z (0, 0, 1) at (0, 0, 25)
extrude "Extrusion38" cut sketch "Esquisse14" along normal blind 8 contours A2 picked at (1.57507, 251.443376) bodies 68
copy_body "Copier/Coller des corps8" bodies 69 68 makes body 70 makes body 71
move_body "Déplacer23" bodies 70 71 to x (1, 0, 0) y (0, 1, 0) z (0, 0, 1) at (-170, 0, 0)
extrude "Extrusion39" add sketch "Esquisse14" along normal blind 3 separate body contours A1 picked at (13.899477, 248.65862) makes body 72
move_body "Déplacer24" bodies 72 to x (1, 0, 0) y (0, 1, 0) z (0, 0, 1) at (0, 0, 33)
copy_body "Copier/Coller des corps9" bodies 72 makes body 73
move_body "Déplacer25" bodies 73 to x (1, 0, 0) y (0, 1, 0) z (0, 0, 1) at (0, 0, -25)
combine "Combiner10" operation cut target body 68 tool bodies 73